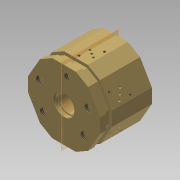
# Autodesk Inventor part: body
Saved by Autodesk Inventor 2014 (Build 180170000, 170)
## iProperties
Created: 2013-10-01
Part Number: body
Material: Generic
Document SubType Name: Modeling
Designer: Admin
Density: 1 g/cm^3
Appearance: Default(1)
Mass: 57.829 g
Surface Area: 134.783 cm^2
Volume: 57.829 cm^3
Author: Admin
Autodesk Inventor part; units mm, degrees
ref_plane "XZ Plane" through (0, 0, 0) normal (0, 1, 0) x (-1, 0, 0)
ref_plane "XY Plane" through (0, 0, 0) normal (0, 0, 1) x (1, 0, 0)
sketch "Sketch1" plane through (0, 0, 0) normal (0, 1, 0) x (-1, 0, 0)
  line L0 (27, 0) -> (13.5, -23.382686)
  line L1 (13.5, -23.382686) -> (-13.5, -23.382686)
  line L2 (-13.5, -23.382686) -> (-27, 0)
  line L3 (-27, 0) -> (-13.5, 23.382686)
  line L4 (-13.5, 23.382686) -> (13.5, 23.382686)
  line L5 (13.5, 23.382686) -> (27, 0)
  point P0 (0, 0)
  point P1 (0, 0)
  dimension "d0" = 27
  constraints: 12 end point, 1 coincident, 13 other
  measures "d0" distance of L0.start point (0, 0)
extrude "body" add sketch "Sketch1" along normal mid plane 35
sketch "Sketch2" plane through (0, -17.5, 0) normal (0, -1, 0) x (1, 0, 0)
  circle A0 centre (0, 0) radius 6.5
  dimension "d4" = 13
  constraints: 1 centre point, 1 coincident
  measures "d4" diameter of A0
extrude "big opening" cut sketch "Sketch2" against normal blind 15
sketch "Sketch3" plane through (0, -2.5, 0) normal (0, -1, 0) x (1, 0, 0)
  circle A0 centre (0, 0) radius 6.5 projected
  circle A1 centre (0, 0) radius 2
  dimension "d7" = 4
  constraints: 1 centre point, 1 coincident
  measures "d7" diameter of A1
extrude "chamber" cut sketch "Sketch3" against normal blind 5 contours A1
sketch "Sketch4" plane through (0, 17.5, 0) normal (0, 1, 0) x (1, 0, 0)
  circle A0 centre (0, 0) radius 4
  dimension "d10" = 8
  constraints: 1 centre point, 1 coincident
  measures "d10" diameter of A0
extrude "small opening" cut sketch "Sketch4" against normal blind 15
sketch "Sketch5" plane through (-13.5, 17.5, 23.382686) normal (0, 0, 1) x (1, 0, 0)
  circle A0 centre (13.5, -17.5) radius 0.75
  dimension "d13" = 1.5
  constraints: 1 centre point, 1 coincident
  measures "d13" diameter of A0
extrude "bore to chamber - NC odor valve" cut sketch "Sketch5" against normal blind 21.75
sketch "Sketch6" plane through (-13.5, 17.5, 23.382686) normal (0, 0, 1) x (1, 0, 0)
  circle A0 centre (16.253961, -19.09) radius 0.75
  line L0 (27, -35) -> (0, -35)
  line L1 (16.220757, -17.5) -> (16.880651, -17.5) construction
  circle A1 centre (13.5, -17.5) radius 0.75
  line L2 (0, 0) -> (0, -35)
  line L3 (9.194703, -17.5) -> (21.882149, -17.5) construction
  line L4 (21.882149, -17.5) -> (9.194703, -17.5) construction
  line L5 (9.194703, -17.5) -> (21.413805, -17.5) construction
  line L6 (13.5, -17.5) -> (19.822818, -21.150481) construction
  line L7 (13.5, -17.5) -> (20.800962, -17.5) construction
  dimension "d16" = 1.5
  dimension "d287" = 3.18
  dimension "d353" = 30
  constraints: 12 end point, 2 horizontal, 1 centre point, 1 collinear, 1 equal length, 1 parallel, 1 perpendicular
  measures "d16" diameter of A0
  measures "d287" distance of L6.start A0.centre
  measures "d353" angle of L6 L7
extrude "odor in - COM odor valve" cut sketch "Sketch6" against normal blind 6 contours A0
sketch "Sketch7" plane through (-13.5, 17.5, 23.382686) normal (0, 0, 1) x (1, 0, 0)
  circle A0 centre (19.007922, -20.68) radius 0.75
  circle A1 centre (16.253961, -19.09) radius 0.75
  circle A2 centre (13.5, -17.5) radius 0.75
  line L0 (13.5, -17.5) -> (16.253961, -19.09) construction
  line L1 (16.253961, -19.09) -> (20.402741, -21.485299) construction
  dimension "d20" = 1.5
  dimension "d292" = 3.18
  constraints: 4 end point, 1 centre point, 1 collinear
  measures "d20" diameter of A0
  measures "d292" distance of A0.centre L0.end
extrude "waste - NO odor valve" cut sketch "Sketch7" against normal blind 6 contours A0
sketch "Sketch14" plane through (0, -17.5, 0) normal (0, -1, 0) x (1, 0, 0)
  line L0 (13.5, 23.382686) -> (-13.5, 23.382686)
  circle A0 centre (2.753961, 17.382686) radius 2.5
  line L1 (-8, -23.382686) -> (8, -23.382686)
  line L2 (9.876388, 17.382686) -> (-9.588253, 17.382686) construction
  line L3 (2.003961, 17.382686) -> (3.503961, 17.382686)
  point P0 (0, 17.382686)
  point P1 (0, 17.382686)
  point P2 (3.18, 17.382686)
  dimension "d46" = 5
  dimension "d47" = 6
  constraints: 2 end point, 2 point on line, 1 centre point, 1 coincident, 1 midpoint, 1 parallel
  measures "d46" diameter of A0
  measures "d47" distance from line of L0 A0.centre
sketch "Sketch24" plane through (0, 17.5, 0) normal (0, 1, 0) x (1, 0, 0)
  line L0 (-13.5, -23.382686) -> (13.5, -23.382686)
  circle A0 centre (5.507922, -17.382686) radius 2.5
  line L1 (6.257922, -17.382686) -> (4.757922, -17.382686)
  point P0 (6.36, -17.382686)
  dimension "d80" = 5
  dimension "d81" = 6
  constraints: 1 centre point, 1 midpoint
  measures "d80" diameter of A0
  measures "d81" distance from line of L0 A0.centre
sketch "Sketch27" plane through (-13.5, 17.5, 23.382686) normal (0, 0, 1) x (1, 0, 0)
  circle A0 centre (16.253961, -19.09) radius 0.75
  circle A1 centre (19.007922, -20.68) radius 0.75
  circle A2 centre (13.5, -17.5) radius 0.75
  line L0 (13.5, -17.5) -> (19.007922, -20.68) construction
  line L1 (19.007922, -20.68) -> (16.253961, -19.09) construction
  line L2 (16.253961, -19.09) -> (21.087831, -10.717491) construction
  line L3 (21.087831, -10.717491) -> (11.918516, -26.599211) construction
  point P0 (19.416461, -13.612389)
  point P1 (13.091461, -24.567611)
  dimension "d290" = 6.325
  dimension "d291" = 6.325
  dimension "d354" = 90
  constraints: 8 end point, 1 collinear, 1 perpendicular
  measures "d290" distance of L1.end point (13.091, -24.568)
  measures "d291" distance of L1.end point (19.416, -13.612)
  measures "d354" angle of L1 L2
hole "valve screws" at (5.916461, 3.887611, 23.382686) at (-0.408539, -7.067611, 23.382686) direction (0, 0, -1) diameter 1.567 depth 4 tip angle 118 thread size "M2x0.4" class "6H" standard "ISO Metric profile"
pattern_circular "odor valves" count 3 over 120 about axis through (0, -10, 0) along (0, 1, 0) of "bore to chamber - NC odor valve", "odor in - COM odor valve", "waste - NO odor valve", "valve screws"
chamfer "Chamfer1" distance 5.5 angle 45 6 edges at (13.5, 0, 23.3827) (27, 0, 0) (-13.5, 0, 23.3827) (-27, 0, 0) (13.5, 0, -23.3827) (-13.5, 0, -23.3827)
sketch "Sketch32" plane through (-8, -17.5, 23.382686) normal (0, 0, 1) x (1, 0, 0)
  line L0 (8, 20.68) -> (8, -12.017365)
  line L1 (1.675, 17.5) -> (14.325, 17.5)
  line L2 (0, 8) -> (0, 4)
  line L3 (16, 8) -> (16, 4)
  line L4 (0, 35) -> (16, 35)
  line L5 (0, 8) -> (16, 8)
  line L6 (0, 0) -> (0, 35)
  line L7 (16, 4) -> (0, 4)
  line L8 (16, 0) -> (0, 0)
  point P0 (8, 8.546288)
  point P1 (8, 5)
  point P2 (8, 17.5)
  point P3 (8, 14.32)
  dimension "d296" = 4
  dimension "d362" = 4
  constraints: 12 end point, 2 point on line, 1 parallel, 1 perpendicular
  measures "d296" distance of L2.start L2.end
  measures "d362" distance between parallel lines of L8 L7
sketch "Sketch33" plane through (16.25, -17.5, 18.619546) normal (0.5, 0, 0.8660254) x (0.8660254, 0, -0.5)
  line L0 (-9.526279, 8) -> (0, 8)
  line L1 (0, 8) -> (0, 4)
  line L2 (0, 4) -> (-9.526279, 4)
  line L3 (-9.526279, 8) -> (-9.526279, 4)
  line L4 (-9.526279, 0) -> (0, 0)
  dimension "d299" = 4
  dimension "d363" = 4
  constraints: 8 end point
  measures "d299" distance between parallel lines of L2 L0
  measures "d363" distance between parallel lines of L4 L2
extrude "cable 1" cut sketch "Sketch32" against normal blind 2 contours L5 L3 L7 L0 | L0 L7 L2 L5
extrude "cable 2" cut sketch "Sketch33" against normal blind 2
pattern_circular "cable path" count 6 over 360 about axis through (0, -10, 0) along (0, 1, 0) of "cable 1", "cable 2"
sketch "Sketch38" plane through (0, 0, 0) normal (1, 0, 0) x (0, 1, 0)
  line L0 (-15, 6.8) -> (-15, 2.528384) construction
  line L1 (-5, 6.8) -> (-5, 2.528384) construction
  line L2 (15, 4.3) -> (15, 2.3) construction
  line L3 (5, 4.3) -> (5, 2.3) construction
  line L4 (-15.5, 2.028384) -> (-14.5, 2.028384)
  line L5 (-14.5, 2.028384) -> (-14.5, 7.3)
  line L6 (-14.5, 7.3) -> (-15.5, 7.3)
  line L7 (-15.5, 7.3) -> (-15.5, 2.028384)
  line L8 (-15.5, 2.028384) -> (-14.5, 7.3) construction
  line L9 (-14.5, 2.028384) -> (-15.5, 7.3) construction
  line L10 (-5.5, 2.028384) -> (-4.5, 2.028384)
  line L11 (-4.5, 7.3) -> (-5.5, 7.3)
  line L12 (-5.5, 2.028384) -> (-4.5, 7.3) construction
  line L13 (-4.5, 2.028384) -> (-5.5, 7.3) construction
  line L14 (4.5, 1.8) -> (5.5, 1.8)
  line L15 (5.5, 1.8) -> (5.5, 4.8)
  line L16 (5.5, 4.8) -> (4.5, 4.8)
  line L17 (4.5, 4.8) -> (4.5, 1.8)
  line L18 (4.5, 1.8) -> (5.5, 4.8) construction
  line L19 (5.5, 1.8) -> (4.5, 4.8) construction
  line L20 (14.5, 1.8) -> (15.5, 1.8)
  line L21 (15.5, 1.8) -> (15.5, 4.8)
  line L22 (15.5, 4.8) -> (14.5, 4.8)
  line L23 (14.5, 4.8) -> (14.5, 1.8)
  line L24 (14.5, 1.8) -> (15.5, 4.8) construction
  line L25 (15.5, 1.8) -> (14.5, 4.8) construction
  line L26 (-5.5, 7.3) -> (-5.5, 2.028384)
  line L27 (-4.5, 2.028384) -> (-4.5, 7.3)
  line L28 (-24.5, 0) -> (24.5, 0)
  point P0 (0, 0)
  point P1 (-15, 4.664192)
  point P2 (-5, 4.664192)
  point P3 (15, 3.3)
  point P4 (5, 3.3)
  constraints: 64 end point, 12 midpoint, 9 parallel, 4 horizontal, 3 perpendicular
extrude "Extrusion30" cut sketch "Sketch14" against normal blind 2
sketch "Sketch39" plane through (2.753961, -15.5, 17.382686) normal (0, -1, 0) x (1, 0, 0)
  circle A0 centre (0, 0) radius 2.5 projected
  circle A1 centre (0, 0) radius 0.75
  point P0 (-2.753961, -17.382686)
  dimension "d250" = 1.5
  constraints: 1 centre point, 1 coincident
  measures "d250" diameter of A1
extrude "Extrusion31" cut sketch "Sketch39" against normal blind 14.66 contours A1
extrude "Extrusion32" cut sketch "Sketch24" against normal blind 2
sketch "Sketch40" plane through (5.507922, 15.5, 17.382686) normal (0, 1, 0) x (1, 0, 0)
  circle A0 centre (0, 0) radius 2.5 projected
  circle A1 centre (0, 0) radius 0.75
  point P0 (-5.507922, 17.382686)
  dimension "d257" = 1.5
  constraints: 1 centre point, 1 coincident
  measures "d257" diameter of A1
extrude "Extrusion33" cut sketch "Sketch40" against normal blind 19.43 contours A1
pattern_circular "Circular Pattern9" count 3 over 120 about axis through (0, -10, 0) along (0, 1, 0) of "Extrusion30", "Extrusion31", "Extrusion32", "Extrusion33"
sketch "Sketch43" plane through (-24.25, -17.5, 4.76314) normal (-0.8660254, 0, 0.5) x (0.5, 0, 0.8660254)
  circle A0 centre (8, 17.5) radius 0.75
  circle A1 centre (8.408539, 24.567611) radius 0.7835
  circle A2 centre (2.083539, 13.612389) radius 0.7835
  constraints: 3 centre point
hole "Hole6" at (-20.04573, 7.067611, 12.045148) at (-23.20823, -3.887611, 6.567538) direction (0.8660254, 0, -0.5) diameter 1.567 depth 4 tip angle 118 thread size "M2x0.4" class "6H" standard "ISO Metric profile"
sketch "Sketch44" plane through (-24.25, -17.5, 4.76314) normal (-0.8660254, 0, 0.5) x (0.5, 0, 0.8660254)
  circle A0 centre (2.492078, 20.68) radius 0.75
  circle A1 centre (5.246039, 19.09) radius 0.75
  point P0 (8, 17.5)
  constraints: 2 centre point, 1 other
extrude "Extrusion34" cut sketch "Sketch44" against normal blind 6
sketch "Sketch45" plane through (0, 17.5, 0) normal (0, 1, 0) x (1, 0, 0)
  line L0 (-17.432808, -4.570862) -> (-18.182808, -3.271824)
  line L1 (-16.055828, -6.955862) -> (-16.805828, -5.656824)
  circle A0 centre (-17.807808, -3.921343) radius 2.5
  point P0 (-16.430828, -6.306343)
  constraints: 2 midpoint, 1 centre point
extrude "Extrusion35" cut sketch "Sketch45" against normal blind 2
sketch "Sketch46" plane through (-17.807808, 15.5, 3.921343) normal (0, 1, 0) x (1, 0, 0)
  circle A0 centre (0, 0) radius 2.5 projected
  circle A1 centre (0, 0) radius 0.75
  point P0 (17.807808, 3.921343)
  dimension "d314" = 1.5
  constraints: 1 centre point, 1 coincident
  measures "d314" diameter of A1
extrude "Extrusion36" cut sketch "Sketch46" against normal blind 13.07 contours A1
sketch "Sketch47" plane through (0, -17.5, 0) normal (0, -1, 0) x (1, 0, 0)
  line L0 (-16.805828, 5.656824) -> (-16.055828, 6.955862)
  circle A0 centre (-16.430828, 6.306343) radius 2.5
  constraints: 1 centre point, 1 midpoint
extrude "Extrusion37" cut sketch "Sketch47" against normal blind 2
sketch "Sketch48" plane through (-16.430828, -15.5, 6.306343) normal (0, -1, 0) x (1, 0, 0)
  circle A0 centre (0, 0) radius 2.5 projected
  circle A1 centre (0, 0) radius 0.75
  point P0 (16.430828, -6.306343)
  dimension "d319" = 1.5
  constraints: 1 centre point, 1 coincident
  measures "d319" diameter of A1
extrude "Extrusion38" cut sketch "Sketch48" against normal blind 17.84 contours A1
chamfer "Chamfer2" distance 0.5 angle 45 2 edges at (-6.5, -17.5, 0) (-4, 17.5, 0)
revolve "Revolution2" cut sketch "Sketch38" angle 360 about axis through (0, -10, 0) along (0, 1, 0)
sketch "Sketch49" plane through (-24.25, -17.5, 4.76314) normal (-0.8660254, 0, 0.5) x (0.5, 0, 0.8660254)
  circle A0 centre (8, 17.5) radius 0.75
  point P0 (8, 17.5)
  dimension "d326" = 1.5
  constraints: 1 centre point, 1 coincident
  measures "d326" diameter of A0
extrude "Extrusion39" cut sketch "Sketch49" against normal blind 21.75
pattern_circular "Circular Pattern12" count 2 over 60 about axis through (0, -10, 0) along (0, -1, 0) of "Hole6", "Extrusion39", "Extrusion34", "Extrusion35", "Extrusion36", "Extrusion37", "Extrusion38"
thread "Thread15" size "M5x0.8" class "6H" standard "ANSI Metric M Profile" full length
thread "Thread16" size "M5x0.8" class "6H" standard "ANSI Metric M Profile" full length
thread "Thread17" size "M5x0.8" class "6H" standard "ANSI Metric M Profile" full length
thread "Thread18" size "M5x0.8" class "6H" standard "ANSI Metric M Profile" full length
thread "Thread19" size "M5x0.8" class "6H" standard "ANSI Metric M Profile" full length
thread "Thread20" size "M5x0.8" class "6H" standard "ANSI Metric M Profile" full length
thread "Thread21" size "M5x0.8" class "6H" standard "ANSI Metric M Profile" full length
thread "Thread22" size "M5x0.8" class "6H" standard "ANSI Metric M Profile" full length
thread "Thread23" size "M5x0.8" class "6H" standard "ANSI Metric M Profile" full length
thread "Thread24" size "M5x0.8" class "6H" standard "ANSI Metric M Profile" full length
sketch "Sketch51" plane through (8, -17.5, -23.382686) normal (0, 0, -1) x (-1, 0, 0)
  circle A0 centre (8, 27) radius 1.621071
  circle A1 centre (8.008091, 17) radius 1.621071
  line L0 (0, 35) -> (16, 35)
  point P0 (8, 17.5)
  dimension "d366" = 10
  dimension "d367" = 8
  constraints: 2 centre point
  measures "d366" distance of A0.centre A1.centre
  measures "d367" distance from line of L0 A0.centre
hole "Hole8" at (0, 9.5, -23.382686) at (-0.008091, -0.5, -23.382686) direction (0, 0, 1) diameter 4.134 depth 8 tip angle 118 thread size "M5x0.8" class "6H" standard "ISO Metric profile"
body "Solid1"
